New Bottom Plate_v4 (Autodesk Fusion 360 design; units mm, degrees)
Autodesk Fusion 360 part; units mm, degrees
note: some values were not read from the file. Set by a fixed rule: which sketch regions a step uses.
sketch "Reference" plane through (0, 0, 0) normal (0, 0, 1) x (1, 0, 0)
  line L0 (298.2751, -95.25) -> (298.2751, -113.3)
  line L1 (298.275, 1) -> (298.275, -57.15)
  line L2 (298.275, -57.15) -> (298.275, -57.15)
  line L3 (304.5217, -115.3) -> (303.775, 3)
  line L4 (179.47, 0) -> (290.235, 0)
  line L5 (290.2351, -112.3) -> (230.642, -112.3)
  line L6 (290.235, 1) -> (298.275, 1)
  line L7 (290.235, 0) -> (298.275, 0)
  line L8 (290.2351, -112.3) -> (298.2751, -112.3)
  arc A0 (302.0217, -117.8) -> (304.5217, -115.3) centre (302.0374, -115.3157) ccw
  line L9 (298.2751, -57.15) -> (298.2751, -74.2)
  line L10 (171.43, 0) -> (171.43, 1)
  line L11 (230.642, -112.3) -> (230.642, -113.3)
  line L12 (222.602, -113.3) -> (222.602, -112.3)
  arc A1 (303.775, 3) -> (301.275, 5.5) centre (301.275, 3) ccw
  line L13 (-28.337, -112.3) -> (-29.3375, -112.3)
  line L14 (-28.3375, 1.5) -> (-28.3375, 3)
  line L15 (-28.337, 1.5) -> (-6.3413, 1.5)
  line L16 (230.642, -112.3) -> (230.642, -113.3)
  line L17 (230.642, -113.3) -> (222.602, -113.3)
  line L18 (-36.12, -117.7958) -> (-31.338, -117.8)
  line L19 (222.602, -113.3) -> (222.602, -112.3)
  line L20 (-28.337, -113.3) -> (-28.337, -112.3)
  line L21 (-29.3375, -113.3) -> (-29.338, -113.3)
  arc A2 (-38.6178, -115.2937) -> (-36.12, -117.7958) centre (-36.1178, -115.2958) ccw
  line L22 (57.336, -112.3) -> (-20.297, -112.3)
  line L23 (8.02, 1) -> (8.02, 0)
  line L24 (-29.3375, -112.3) -> (-29.3375, -113.3)
  line L25 (-33.0995, -112.3) -> (-33.0995, 1.5)
  line L26 (-29.338, -112.3) -> (-33.0995, -112.3)
  line L27 (57.336, -113.3) -> (57.336, -112.3)
  line L28 (-20.297, -113.3) -> (-28.337, -113.3)
  line L29 (-29.338, -113.3) -> (-29.338, -112.3)
  line L30 (-20.297, -112.3) -> (-20.297, -113.3)
  line L31 (301.275, 5.5) -> (-36.0995, 5.5)
  line L32 (-38.5995, -94.25) -> (-38.6178, -115.2937)
  line L33 (298.2751, -76.2) -> (298.2751, -93.25)
  line L34 (298.275, -95.25) -> (298.275, -95.25)
  line L35 (298.275, -76.2) -> (298.275, -76.2)
  line L36 (-6.3413, 1.5) -> (-6.3413, 0)
  line L37 (-38.5995, 3) -> (-38.5995, -94.25)
  arc A3 (303.775, 3) -> (301.275, 5.5) centre (301.275, 3) ccw
  line L38 (298.2751, -74.2) -> (298.275, -74.2)
  line L39 (-28.337, 3) -> (-28.337, 1.5)
  line L40 (-33.0995, 1.5) -> (-28.3375, 1.5)
  line L41 (-0.02, 0) -> (-0.02, 1)
  arc A4 (-36.0995, 5.5) -> (-38.5995, 3) centre (-36.0995, 3) ccw
  line L42 (-31.338, -117.8) -> (302.0217, -117.8)
  line L43 (-6.3413, 0) -> (-0.02, 0)
  line L44 (298.275, -57.15) -> (298.275, -57.15)
  line L45 (-0.02, 1) -> (8.02, 1)
  line L46 (8.02, 0) -> (171.43, 0)
  line L47 (-28.3375, 3) -> (-28.337, 3)
  line L48 (290.235, 0) -> (290.235, 1)
  line L49 (290.235, 1) -> (298.275, 1)
  line L50 (298.2751, -57.15) -> (298.2751, -74.2)
  line L51 (298.275, 1) -> (298.275, -57.15)
  line L52 (222.602, -112.3) -> (65.376, -112.3)
  line L53 (-33.0995, -112.3) -> (-33.0995, 1.5)
  line L54 (301.275, 5.5) -> (-36.0995, 5.5)
  line L55 (-31.338, -117.8) -> (302.0217, -117.8)
  line L56 (57.336, -112.3) -> (-20.297, -112.3)
  line L57 (8.02, 0) -> (171.43, 0)
  line L58 (290.2351, -112.3) -> (230.642, -112.3)
  line L59 (298.2751, -95.25) -> (298.2751, -113.3)
  line L60 (298.275, -76.2) -> (298.275, -76.2)
  line L61 (298.275, -74.2) -> (298.275, -76.2)
  line L62 (298.2751, -76.2) -> (298.2751, -93.25)
  line L63 (298.2751, -93.25) -> (298.275, -93.25)
  line L64 (298.275, -93.25) -> (298.275, -95.25)
  line L65 (290.2351, -113.3) -> (290.2351, -112.3)
  arc A5 (302.0217, -117.8) -> (304.5217, -115.3) centre (302.0374, -115.3157) ccw
  line L66 (179.47, 0) -> (290.235, 0)
  line L67 (298.2751, -113.3) -> (290.2351, -113.3)
  line L68 (304.5217, -115.3) -> (303.775, 3)
  line L69 (298.275, -95.25) -> (298.275, -95.25)
  line L70 (57.336, -113.3) -> (57.336, -112.3)
  line L71 (65.376, -113.3) -> (57.336, -113.3)
  line L72 (-29.338, -113.3) -> (-29.338, -112.3)
  line L73 (-6.3413, 1.5) -> (-6.3413, 0)
  line L74 (-29.3375, -113.3) -> (-29.338, -113.3)
  line L75 (-29.3375, -112.3) -> (-29.3375, -113.3)
  line L76 (-28.3375, 1.5) -> (-28.3375, 3)
  line L77 (-28.337, 1.5) -> (-6.3413, 1.5)
  line L78 (-28.337, -112.3) -> (-29.3375, -112.3)
  line L79 (-28.337, -113.3) -> (-28.337, -112.3)
  line L80 (-28.3375, 3) -> (-28.337, 3)
  line L81 (-20.297, -113.3) -> (-28.337, -113.3)
  line L82 (65.376, -112.3) -> (65.376, -113.3)
  line L83 (-20.297, -112.3) -> (-20.297, -113.3)
  line L84 (-29.338, -112.3) -> (-33.0995, -112.3)
  line L85 (8.02, 1) -> (8.02, 0)
  line L86 (-28.337, 3) -> (-28.337, 1.5)
  arc A6 (-38.6178, -115.2937) -> (-36.12, -117.7958) centre (-36.1178, -115.2958) ccw
  line L87 (-38.5995, -94.25) -> (-38.6178, -115.2937)
  line L88 (-38.5995, 3) -> (-38.5995, -94.25)
  line L89 (-0.02, 0) -> (-0.02, 1)
  line L90 (-33.0995, 1.5) -> (-28.3375, 1.5)
  line L91 (-6.3413, 0) -> (-0.02, 0)
  arc A7 (-36.0995, 5.5) -> (-38.5995, 3) centre (-36.0995, 3) ccw
  line L92 (-0.02, 1) -> (8.02, 1)
  line L93 (-36.12, -117.7958) -> (-31.338, -117.8)
  line L94 (298.275, -93.25) -> (298.275, -95.25)
  line L95 (298.2751, -113.3) -> (290.2351, -113.3)
  line L96 (290.2351, -113.3) -> (290.2351, -112.3)
  line L97 (298.2751, -93.25) -> (298.275, -93.25)
  line L98 (298.275, -74.2) -> (298.275, -76.2)
  line L99 (298.2751, -74.2) -> (298.275, -74.2)
  line L100 (290.235, 0) -> (290.235, 1)
  line L101 (179.47, 1) -> (179.47, 0)
  line L102 (230.642, -113.3) -> (222.602, -113.3)
  line L103 (179.47, 1) -> (179.47, 0)
  line L104 (171.43, 1) -> (179.47, 1)
  line L105 (222.602, -112.3) -> (65.376, -112.3)
  line L106 (65.376, -112.3) -> (65.376, -113.3)
  line L107 (65.376, -113.3) -> (57.336, -113.3)
  line L108 (171.43, 0) -> (171.43, 1)
  line L109 (171.43, 1) -> (179.47, 1)
  dimension "d29" = 5.5
  dimension "d30" = 5.5
  dimension "d31" = 6.2339
  dimension "d32" = 5.5125
  dimension "d33" = 5.5
  dimension "d34" = 6.2276
  dimension "d35" = 5.5188
  constraint coincident L5.start L8.start
  constraint perpendicular L0 L8
  constraint coincident L8.end L59
  constraint coincident L4.end L7.start
  constraint perpendicular L7 L48
  constraint coincident L7.end L51
  measures "d29" distance of L42 L58
  measures "d30" distance of L4 L31
  measures "d31" distance of L0.end L3
  measures "d32" distance of L1.start L3
  measures "d33" distance of L25 L37
  measures "d34" distance of L8.end L3
  measures "d35" distance of L7.end L68
sketch "FlatPlateSketch" plane through (0, 0, 0) normal (0, 0, 1) x (1, 0, 0)
  line L0 (298.2751, -95.25) -> (298.2751, -113.3)
  line L1 (298.275, 1) -> (298.275, -57.15)
  line L2 (298.275, -57.15) -> (298.275, -57.15)
  line L3 (304.5217, -115.3) -> (303.775, 3)
  line L4 (179.47, 0) -> (290.235, 0)
  line L5 (290.2351, -112.3) -> (230.642, -112.3)
  line L6 (290.235, 1) -> (298.275, 1)
  line L7 (290.235, 0) -> (298.275, 0)
  line L8 (290.2351, -112.3) -> (298.2751, -112.3)
  arc A0 (302.0217, -117.8) -> (304.5217, -115.3) centre (302.0374, -115.3157) ccw
  line L9 (298.2751, -57.15) -> (298.2751, -74.2)
  line L10 (171.43, 0) -> (171.43, 1)
  line L11 (230.642, -112.3) -> (230.642, -113.3)
  line L12 (222.602, -113.3) -> (222.602, -112.3)
  arc A1 (303.775, 3) -> (301.275, 5.5) centre (301.275, 3) ccw
  line L13 (-28.337, -112.3) -> (-29.3375, -112.3)
  line L14 (-28.3375, 1.5) -> (-28.3375, 3)
  line L15 (-28.337, 1.5) -> (-6.3413, 1.5)
  line L16 (230.642, -112.3) -> (230.642, -113.3)
  line L17 (230.642, -113.3) -> (222.602, -113.3)
  line L18 (-36.12, -117.7958) -> (-31.338, -117.8)
  line L19 (222.602, -113.3) -> (222.602, -112.3)
  line L20 (-28.337, -113.3) -> (-28.337, -112.3)
  line L21 (-29.3375, -113.3) -> (-29.338, -113.3)
  arc A2 (-38.6178, -115.2937) -> (-36.12, -117.7958) centre (-36.1178, -115.2958) ccw
  line L22 (57.336, -112.3) -> (-20.297, -112.3)
  line L23 (8.02, 1) -> (8.02, 0)
  line L24 (-29.3375, -112.3) -> (-29.3375, -113.3)
  line L25 (-33.0995, -112.3) -> (-33.0995, 1.5)
  line L26 (-29.338, -112.3) -> (-33.0995, -112.3)
  line L27 (57.336, -113.3) -> (57.336, -112.3)
  line L28 (-20.297, -113.3) -> (-28.337, -113.3)
  line L29 (-29.338, -113.3) -> (-29.338, -112.3)
  line L30 (-20.297, -112.3) -> (-20.297, -113.3)
  line L31 (301.275, 5.5) -> (-36.0995, 5.5)
  line L32 (-38.5995, -94.25) -> (-38.6178, -115.2937)
  line L33 (298.2751, -76.2) -> (298.2751, -93.25)
  line L34 (298.275, -95.25) -> (298.275, -95.25)
  line L35 (298.275, -76.2) -> (298.275, -76.2)
  line L36 (-6.3413, 1.5) -> (-6.3413, 0)
  line L37 (-38.5995, 3) -> (-38.5995, -94.25)
  arc A3 (303.775, 3) -> (301.275, 5.5) centre (301.275, 3) ccw
  line L38 (298.2751, -74.2) -> (298.275, -74.2)
  line L39 (-28.337, 3) -> (-28.337, 1.5)
  line L40 (-33.0995, 1.5) -> (-28.3375, 1.5)
  line L41 (-0.02, 0) -> (-0.02, 1)
  arc A4 (-36.0995, 5.5) -> (-38.5995, 3) centre (-36.0995, 3) ccw
  line L42 (-31.338, -117.8) -> (302.0217, -117.8)
  line L43 (-6.3413, 0) -> (-0.02, 0)
  line L44 (298.275, -57.15) -> (298.275, -57.15)
  line L45 (-0.02, 1) -> (8.02, 1)
  line L46 (8.02, 0) -> (171.43, 0)
  line L47 (-28.3375, 3) -> (-28.337, 3)
  line L48 (290.235, 0) -> (290.235, 1)
  line L49 (290.235, 1) -> (298.275, 1)
  line L50 (298.2751, -57.15) -> (298.2751, -74.2)
  line L51 (298.275, 1) -> (298.275, -57.15)
  line L52 (222.602, -112.3) -> (65.376, -112.3)
  line L53 (-33.0995, -112.3) -> (-33.0995, 1.5)
  line L54 (301.275, 5.5) -> (-36.0995, 5.5)
  line L55 (-31.338, -117.8) -> (302.0217, -117.8)
  line L56 (57.336, -112.3) -> (-20.297, -112.3)
  line L57 (8.02, 0) -> (171.43, 0)
  line L58 (290.2351, -112.3) -> (230.642, -112.3)
  line L59 (298.2751, -95.25) -> (298.2751, -113.3)
  line L60 (298.275, -76.2) -> (298.275, -76.2)
  line L61 (298.275, -74.2) -> (298.275, -76.2)
  line L62 (298.2751, -76.2) -> (298.2751, -93.25)
  line L63 (298.2751, -93.25) -> (298.275, -93.25)
  line L64 (298.275, -93.25) -> (298.275, -95.25)
  line L65 (290.2351, -113.3) -> (290.2351, -112.3)
  arc A5 (302.0217, -117.8) -> (304.5217, -115.3) centre (302.0374, -115.3157) ccw
  line L66 (179.47, 0) -> (290.235, 0)
  line L67 (298.2751, -113.3) -> (290.2351, -113.3)
  line L68 (304.5217, -115.3) -> (303.775, 3)
  line L69 (298.275, -95.25) -> (298.275, -95.25)
  line L70 (57.336, -113.3) -> (57.336, -112.3)
  line L71 (65.376, -113.3) -> (57.336, -113.3)
  line L72 (-29.338, -113.3) -> (-29.338, -112.3)
  line L73 (-6.3413, 1.5) -> (-6.3413, 0)
  line L74 (-29.3375, -113.3) -> (-29.338, -113.3)
  line L75 (-29.3375, -112.3) -> (-29.3375, -113.3)
  line L76 (-28.3375, 1.5) -> (-28.3375, 3)
  line L77 (-28.337, 1.5) -> (-6.3413, 1.5)
  line L78 (-28.337, -112.3) -> (-29.3375, -112.3)
  line L79 (-28.337, -113.3) -> (-28.337, -112.3)
  line L80 (-28.3375, 3) -> (-28.337, 3)
  line L81 (-20.297, -113.3) -> (-28.337, -113.3)
  line L82 (65.376, -112.3) -> (65.376, -113.3)
  line L83 (-20.297, -112.3) -> (-20.297, -113.3)
  line L84 (-29.338, -112.3) -> (-33.0995, -112.3)
  line L85 (8.02, 1) -> (8.02, 0)
  line L86 (-28.337, 3) -> (-28.337, 1.5)
  arc A6 (-38.6178, -115.2937) -> (-36.12, -117.7958) centre (-36.1178, -115.2958) ccw
  line L87 (-38.5995, -94.25) -> (-38.6178, -115.2937)
  line L88 (-38.5995, 3) -> (-38.5995, -94.25)
  line L89 (-0.02, 0) -> (-0.02, 1)
  line L90 (-33.0995, 1.5) -> (-28.3375, 1.5)
  line L91 (-6.3413, 0) -> (-0.02, 0)
  arc A7 (-36.0995, 5.5) -> (-38.5995, 3) centre (-36.0995, 3) ccw
  line L92 (-0.02, 1) -> (8.02, 1)
  line L93 (-36.12, -117.7958) -> (-31.338, -117.8)
  line L94 (298.275, -93.25) -> (298.275, -95.25)
  line L95 (298.2751, -113.3) -> (290.2351, -113.3)
  line L96 (290.2351, -113.3) -> (290.2351, -112.3)
  line L97 (298.2751, -93.25) -> (298.275, -93.25)
  line L98 (298.275, -74.2) -> (298.275, -76.2)
  line L99 (298.2751, -74.2) -> (298.275, -74.2)
  line L100 (290.235, 0) -> (290.235, 1)
  line L101 (179.47, 1) -> (179.47, 0)
  line L102 (230.642, -113.3) -> (222.602, -113.3)
  line L103 (179.47, 1) -> (179.47, 0)
  line L104 (171.43, 1) -> (179.47, 1)
  line L105 (222.602, -112.3) -> (65.376, -112.3)
  line L106 (65.376, -112.3) -> (65.376, -113.3)
  line L107 (65.376, -113.3) -> (57.336, -113.3)
  line L108 (171.43, 0) -> (171.43, 1)
  line L109 (171.43, 1) -> (179.47, 1)
  dimension "d36" = 5.5
  dimension "d37" = 5.5
  dimension "d38" = 6.2339
  dimension "d39" = 5.5125
  dimension "d40" = 5.5
  dimension "d41" = 6.2276
  dimension "d42" = 5.5188
  constraint coincident L5.start L8.start
  constraint perpendicular L0 L8
  constraint coincident L8.end L59
  constraint coincident L4.end L7.start
  constraint perpendicular L7 L48
  constraint coincident L7.end L51
  measures "d36" distance of L42 L58
  measures "d37" distance of L4 L31
  measures "d38" distance of L0.end L3
  measures "d39" distance of L1.start L3
  measures "d40" distance of L25 L37
  measures "d41" distance of L8.end L3
  measures "d42" distance of L7.end L68
sketch "LipSketch" plane through (0, 0, 0) normal (0, 0, 1) x (1, 0, 0)
  line L0 (298.2751, -95.25) -> (298.2751, -113.3)
  line L1 (298.275, 1) -> (298.275, -57.15)
  line L2 (298.275, -57.15) -> (298.275, -57.15)
  line L3 (304.5217, -115.3) -> (303.775, 3)
  line L4 (179.47, 0) -> (290.235, 0)
  line L5 (290.2351, -112.3) -> (230.642, -112.3)
  line L6 (290.235, 1) -> (298.275, 1)
  line L7 (290.235, 0) -> (298.275, 0)
  line L8 (290.2351, -112.3) -> (298.2751, -112.3)
  arc A0 (302.0217, -117.8) -> (304.5217, -115.3) centre (302.0374, -115.3157) ccw
  line L9 (298.2751, -57.15) -> (298.2751, -74.2)
  line L10 (171.43, 0) -> (171.43, 1)
  line L11 (230.642, -112.3) -> (230.642, -113.3)
  line L12 (222.602, -113.3) -> (222.602, -112.3)
  arc A1 (303.775, 3) -> (301.275, 5.5) centre (301.275, 3) ccw
  line L13 (-28.337, -112.3) -> (-29.3375, -112.3)
  line L14 (-28.3375, 1.5) -> (-28.3375, 3)
  line L15 (-28.337, 1.5) -> (-6.3413, 1.5)
  line L16 (230.642, -112.3) -> (230.642, -113.3)
  line L17 (230.642, -113.3) -> (222.602, -113.3)
  line L18 (-36.12, -117.7958) -> (-31.338, -117.8)
  line L19 (222.602, -113.3) -> (222.602, -112.3)
  line L20 (-28.337, -113.3) -> (-28.337, -112.3)
  line L21 (-29.3375, -113.3) -> (-29.338, -113.3)
  arc A2 (-38.6178, -115.2937) -> (-36.12, -117.7958) centre (-36.1178, -115.2958) ccw
  line L22 (57.336, -112.3) -> (-20.297, -112.3)
  line L23 (8.02, 1) -> (8.02, 0)
  line L24 (-29.3375, -112.3) -> (-29.3375, -113.3)
  line L25 (-33.0995, -112.3) -> (-33.0995, 1.5)
  line L26 (-29.338, -112.3) -> (-33.0995, -112.3)
  line L27 (57.336, -113.3) -> (57.336, -112.3)
  line L28 (-20.297, -113.3) -> (-28.337, -113.3)
  line L29 (-29.338, -113.3) -> (-29.338, -112.3)
  line L30 (-20.297, -112.3) -> (-20.297, -113.3)
  line L31 (301.275, 5.5) -> (-36.0995, 5.5)
  line L32 (-38.5995, -94.25) -> (-38.6178, -115.2937)
  line L33 (298.2751, -76.2) -> (298.2751, -93.25)
  line L34 (298.275, -95.25) -> (298.275, -95.25)
  line L35 (298.275, -76.2) -> (298.275, -76.2)
  line L36 (-6.3413, 1.5) -> (-6.3413, 0)
  line L37 (-38.5995, 3) -> (-38.5995, -94.25)
  arc A3 (303.775, 3) -> (301.275, 5.5) centre (301.275, 3) ccw
  line L38 (298.2751, -74.2) -> (298.275, -74.2)
  line L39 (-28.337, 3) -> (-28.337, 1.5)
  line L40 (-33.0995, 1.5) -> (-28.3375, 1.5)
  line L41 (-0.02, 0) -> (-0.02, 1)
  arc A4 (-36.0995, 5.5) -> (-38.5995, 3) centre (-36.0995, 3) ccw
  line L42 (-31.338, -117.8) -> (302.0217, -117.8)
  line L43 (-6.3413, 0) -> (-0.02, 0)
  line L44 (298.275, -57.15) -> (298.275, -57.15)
  line L45 (-0.02, 1) -> (8.02, 1)
  line L46 (8.02, 0) -> (171.43, 0)
  line L47 (-28.3375, 3) -> (-28.337, 3)
  line L48 (290.235, 0) -> (290.235, 1)
  line L49 (290.235, 1) -> (298.275, 1)
  line L50 (298.2751, -57.15) -> (298.2751, -74.2)
  line L51 (298.275, 1) -> (298.275, -57.15)
  line L52 (222.602, -112.3) -> (65.376, -112.3)
  line L53 (-33.0995, -112.3) -> (-33.0995, 1.5)
  line L54 (301.275, 5.5) -> (-36.0995, 5.5)
  line L55 (-31.338, -117.8) -> (302.0217, -117.8)
  line L56 (57.336, -112.3) -> (-20.297, -112.3)
  line L57 (8.02, 0) -> (171.43, 0)
  line L58 (290.2351, -112.3) -> (230.642, -112.3)
  line L59 (298.2751, -95.25) -> (298.2751, -113.3)
  line L60 (298.275, -76.2) -> (298.275, -76.2)
  line L61 (298.275, -74.2) -> (298.275, -76.2)
  line L62 (298.2751, -76.2) -> (298.2751, -93.25)
  line L63 (298.2751, -93.25) -> (298.275, -93.25)
  line L64 (298.275, -93.25) -> (298.275, -95.25)
  line L65 (290.2351, -113.3) -> (290.2351, -112.3)
  arc A5 (302.0217, -117.8) -> (304.5217, -115.3) centre (302.0374, -115.3157) ccw
  line L66 (179.47, 0) -> (290.235, 0)
  line L67 (298.2751, -113.3) -> (290.2351, -113.3)
  line L68 (304.5217, -115.3) -> (303.775, 3)
  line L69 (298.275, -95.25) -> (298.275, -95.25)
  line L70 (57.336, -113.3) -> (57.336, -112.3)
  line L71 (65.376, -113.3) -> (57.336, -113.3)
  line L72 (-29.338, -113.3) -> (-29.338, -112.3)
  line L73 (-6.3413, 1.5) -> (-6.3413, 0)
  line L74 (-29.3375, -113.3) -> (-29.338, -113.3)
  line L75 (-29.3375, -112.3) -> (-29.3375, -113.3)
  line L76 (-28.3375, 1.5) -> (-28.3375, 3)
  line L77 (-28.337, 1.5) -> (-6.3413, 1.5)
  line L78 (-28.337, -112.3) -> (-29.3375, -112.3)
  line L79 (-28.337, -113.3) -> (-28.337, -112.3)
  line L80 (-28.3375, 3) -> (-28.337, 3)
  line L81 (-20.297, -113.3) -> (-28.337, -113.3)
  line L82 (65.376, -112.3) -> (65.376, -113.3)
  line L83 (-20.297, -112.3) -> (-20.297, -113.3)
  line L84 (-29.338, -112.3) -> (-33.0995, -112.3)
  line L85 (8.02, 1) -> (8.02, 0)
  line L86 (-28.337, 3) -> (-28.337, 1.5)
  arc A6 (-38.6178, -115.2937) -> (-36.12, -117.7958) centre (-36.1178, -115.2958) ccw
  line L87 (-38.5995, -94.25) -> (-38.6178, -115.2937)
  line L88 (-38.5995, 3) -> (-38.5995, -94.25)
  line L89 (-0.02, 0) -> (-0.02, 1)
  line L90 (-33.0995, 1.5) -> (-28.3375, 1.5)
  line L91 (-6.3413, 0) -> (-0.02, 0)
  arc A7 (-36.0995, 5.5) -> (-38.5995, 3) centre (-36.0995, 3) ccw
  line L92 (-0.02, 1) -> (8.02, 1)
  line L93 (-36.12, -117.7958) -> (-31.338, -117.8)
  line L94 (298.275, -93.25) -> (298.275, -95.25)
  line L95 (298.2751, -113.3) -> (290.2351, -113.3)
  line L96 (290.2351, -113.3) -> (290.2351, -112.3)
  line L97 (298.2751, -93.25) -> (298.275, -93.25)
  line L98 (298.275, -74.2) -> (298.275, -76.2)
  line L99 (298.2751, -74.2) -> (298.275, -74.2)
  line L100 (290.235, 0) -> (290.235, 1)
  line L101 (179.47, 1) -> (179.47, 0)
  line L102 (230.642, -113.3) -> (222.602, -113.3)
  line L103 (179.47, 1) -> (179.47, 0)
  line L104 (171.43, 1) -> (179.47, 1)
  line L105 (222.602, -112.3) -> (65.376, -112.3)
  line L106 (65.376, -112.3) -> (65.376, -113.3)
  line L107 (65.376, -113.3) -> (57.336, -113.3)
  line L108 (171.43, 0) -> (171.43, 1)
  line L109 (171.43, 1) -> (179.47, 1)
  line L110 (290.235, 0) -> (290.235, -0.5) construction
  line L111 (298.275, -3.3243) -> (297.775, -3.3243) construction
  line L112 (286.7003, -112.3) -> (286.7003, -111.8) construction
  line L113 (298.2751, -110.893) -> (297.7751, -110.893) construction
  line L114 (286.7003, -111.8) -> (297.7751, -111.8)
  line L115 (297.7751, -110.893) -> (297.7751, -111.8)
  line L116 (297.7751, -110.893) -> (297.7751, -0.5)
  line L117 (290.235, -0.5) -> (297.7751, -0.5)
  line L118 (290.235, -0.5) -> (-27.25, -0.5)
  line L119 (-33.0995, -0.5) -> (-32.5995, -0.5) construction
  line L120 (-32.5995, -0.5) -> (-27.25, -0.5)
  line L121 (-33.0995, -111.8) -> (-32.5995, -111.8) construction
  line L122 (-32.5995, -111.8) -> (-32.5995, -0.5)
  line L123 (286.7003, -111.8) -> (-31.0685, -111.8)
  line L124 (-31.0685, -111.8) -> (-32.5995, -111.8)
  line L125 (-32.5995, -0.5) -> (-30.5995, -0.5)
  line L126 (-30.5995, -0.5) -> (-30.5995, -2.5) construction
  line L127 (-32.5995, -2.5) -> (-32.5995, -0.5)
  line L128 (-32.5995, -111.8) -> (-30.5995, -111.8)
  line L129 (-30.5995, -111.8) -> (-30.5995, -109.8) construction
  line L130 (-30.5995, -109.8) -> (-32.5995, -109.8) construction
  line L131 (-32.5995, -109.8) -> (-32.5995, -111.8)
  line L132 (297.7751, -111.8) -> (295.7751, -111.8)
  line L133 (295.7751, -111.8) -> (295.7751, -109.8) construction
  line L134 (295.7751, -109.8) -> (297.7751, -109.8) construction
  line L135 (297.7751, -109.8) -> (297.7751, -111.8)
  line L136 (297.7751, -0.5) -> (295.7751, -0.5)
  line L137 (295.7751, -0.5) -> (295.7751, -2.5) construction
  line L138 (295.7751, -2.5) -> (297.7751, -2.5) construction
  line L139 (297.7751, -2.5) -> (297.7751, -0.5)
  line L140 (295.7751, -2.5) -> (-30.5995, -2.5)
  line L141 (-30.5995, -2.5) -> (-30.5995, -109.8)
  line L142 (-30.5995, -109.8) -> (295.7751, -109.8)
  line L143 (295.7751, -109.8) -> (295.7751, -2.5)
  dimension "d45" = 5.5
  dimension "d46" = 5.5
  dimension "d47" = 6.2339
  dimension "d48" = 5.5125
  dimension "d49" = 5.5
  dimension "d50" = 6.2276
  dimension "d51" = 5.5188
  dimension "d68" = 0.5
  dimension "d69" = 0.5
  dimension "d70" = 0.5
  dimension "d71" = 0.5
  dimension "d72" = 0.5
  dimension "d73" = 0.5
  dimension "d74" = 2
  dimension "d75" = 2
  dimension "d76" = 2
  dimension "d77" = 2
  dimension "d78" = 2
  dimension "d79" = 2
  dimension "d80" = 2
  dimension "d81" = 2
  constraint coincident L5.start L8.start
  constraint perpendicular L0 L8
  constraint coincident L8.end L59
  constraint coincident L4.end L7.start
  constraint perpendicular L7 L48
  constraint coincident L7.end L51
  constraint perpendicular L7 L110
  constraint coincident L1 L111.start
  constraint perpendicular L1 L111
  constraint coincident L58 L112.start
  constraint perpendicular L58 L112
  constraint coincident L59 L113.start
  constraint perpendicular L59 L113
  constraint perpendicular L0 L114
  constraint perpendicular L113 L115
  constraint perpendicular L6 L116
  constraint perpendicular L110 L117
  constraint perpendicular L25 L118
  constraint coincident L25 L119.start
  constraint perpendicular L25 L119
  constraint parallel L119 L120
  constraint perpendicular L25 L123
  constraint coincident L25 L121.start
  constraint perpendicular L53 L121
  constraint horizontal L125
  constraint vertical L126
  constraint vertical L127
  constraint horizontal L128
  constraint vertical L129
  constraint horizontal L130
  constraint vertical L131
  constraint horizontal L132
  constraint vertical L133
  constraint horizontal L134
  constraint vertical L135
  constraint horizontal L136
  constraint vertical L137
  constraint horizontal L138
  constraint vertical L139
  constraint perpendicular L126 L140
  constraint perpendicular L130 L141
  constraint perpendicular L133 L142
  constraint perpendicular L138 L143
  measures "d45" distance of L42 L58
  measures "d46" distance of L4 L31
  measures "d47" distance of L0.end L3
  measures "d48" distance of L1.start L3
  measures "d49" distance of L25 L37
  measures "d50" distance of L8.end L3
  measures "d51" distance of L7.end L68
  measures "d68" distance of L4.end L110.end
  measures "d69" distance of L111.start L111.end
  measures "d70" distance of L112.start L112.end
  measures "d71" distance of L113.start L113.end
  measures "d72" distance of L119.start L119.end
  measures "d73" distance of L121.start L121.end
  measures "d74" distance of L119.end L125.end
  measures "d75" distance of L119.end L127.start
  measures "d76" distance of L121.end L128.end
  measures "d77" distance of L121.end L130.end
  measures "d78" distance of L114.end L132.end
  measures "d79" distance of L114.end L134.end
  measures "d80" distance of L116.end L136.end
  measures "d81" distance of L116.end L138.end
extrude "Extrude4" add sketch "FlatPlateSketch" against normal blind 1 contours L0 L1 L4 L5 L7 L8 L9 L10 L11 L12 L13 L15 L16 L17 L19 L20 L22 L23 L25 L26 L27 L28 L30 L33 L36 L40 L41 L43 L45 L46 L50 L51 L52 L53 L56 L57 L58 L59 L61 L62 L64 L66 L70 L71 L73 L77 L78 L79 L81 L82 L83 L84 L85 L89 L90 L91 L92 L94 L98 L101 L102 L103 L104 L105 L106 L107 L108 L109 | L0 L8 L59 L65 L67 L95 L96 | L1 L6 L7 L48 L49 L51 L100 | L3 A0 A1 L18 A2 L31 L32 L37 A3 A4 L42 L54 L55 A5 L68 A6 L87 L88 A7 L93
sketch "Sketch8" plane through (0, 0, 0) normal (0, 0, 1) x (1, 0, 0)
  line L0 (298.2751, -95.25) -> (298.2751, -113.3)
  line L1 (298.275, 1) -> (298.275, -57.15)
  line L2 (298.275, -57.15) -> (298.275, -57.15)
  line L3 (304.5217, -115.3) -> (303.775, 3)
  line L4 (179.47, 0) -> (290.235, 0)
  line L5 (290.2351, -112.3) -> (230.642, -112.3)
  line L6 (290.235, 1) -> (298.275, 1)
  line L7 (290.235, 0) -> (298.275, 0)
  line L8 (290.2351, -112.3) -> (298.2751, -112.3)
  arc A0 (302.0217, -117.8) -> (304.5217, -115.3) centre (302.0374, -115.3157) ccw
  line L9 (298.2751, -57.15) -> (298.2751, -74.2)
  line L10 (171.43, 0) -> (171.43, 1)
  line L11 (230.642, -112.3) -> (230.642, -113.3)
  line L12 (222.602, -113.3) -> (222.602, -112.3)
  arc A1 (303.775, 3) -> (301.275, 5.5) centre (301.275, 3) ccw
  line L13 (-28.337, -112.3) -> (-29.3375, -112.3)
  line L14 (-28.3375, 1.5) -> (-28.3375, 3)
  line L15 (-28.337, 1.5) -> (-6.3413, 1.5)
  line L16 (230.642, -112.3) -> (230.642, -113.3)
  line L17 (230.642, -113.3) -> (222.602, -113.3)
  line L18 (-36.12, -117.7958) -> (-31.338, -117.8)
  line L19 (222.602, -113.3) -> (222.602, -112.3)
  line L20 (-28.337, -113.3) -> (-28.337, -112.3)
  line L21 (-29.3375, -113.3) -> (-29.338, -113.3)
  arc A2 (-38.6178, -115.2937) -> (-36.12, -117.7958) centre (-36.1178, -115.2958) ccw
  line L22 (57.336, -112.3) -> (-20.297, -112.3)
  line L23 (8.02, 1) -> (8.02, 0)
  line L24 (-29.3375, -112.3) -> (-29.3375, -113.3)
  line L25 (-33.0995, -112.3) -> (-33.0995, 1.5)
  line L26 (-29.338, -112.3) -> (-33.0995, -112.3)
  line L27 (57.336, -113.3) -> (57.336, -112.3)
  line L28 (-20.297, -113.3) -> (-28.337, -113.3)
  line L29 (-29.338, -113.3) -> (-29.338, -112.3)
  line L30 (-20.297, -112.3) -> (-20.297, -113.3)
  line L31 (301.275, 5.5) -> (-36.0995, 5.5)
  line L32 (-38.5995, -94.25) -> (-38.6178, -115.2937)
  line L33 (298.2751, -76.2) -> (298.2751, -93.25)
  line L34 (298.275, -95.25) -> (298.275, -95.25)
  line L35 (298.275, -76.2) -> (298.275, -76.2)
  line L36 (-6.3413, 1.5) -> (-6.3413, 0)
  line L37 (-38.5995, 3) -> (-38.5995, -94.25)
  arc A3 (303.775, 3) -> (301.275, 5.5) centre (301.275, 3) ccw
  line L38 (298.2751, -74.2) -> (298.275, -74.2)
  line L39 (-28.337, 3) -> (-28.337, 1.5)
  line L40 (-33.0995, 1.5) -> (-28.3375, 1.5)
  line L41 (-0.02, 0) -> (-0.02, 1)
  arc A4 (-36.0995, 5.5) -> (-38.5995, 3) centre (-36.0995, 3) ccw
  line L42 (-31.338, -117.8) -> (302.0217, -117.8)
  line L43 (-6.3413, 0) -> (-0.02, 0)
  line L44 (298.275, -57.15) -> (298.275, -57.15)
  line L45 (-0.02, 1) -> (8.02, 1)
  line L46 (8.02, 0) -> (171.43, 0)
  line L47 (-28.3375, 3) -> (-28.337, 3)
  line L48 (290.235, 0) -> (290.235, 1)
  line L49 (290.235, 1) -> (298.275, 1)
  line L50 (298.2751, -57.15) -> (298.2751, -74.2)
  line L51 (298.275, 1) -> (298.275, -57.15)
  line L52 (222.602, -112.3) -> (65.376, -112.3)
  line L53 (-33.0995, -112.3) -> (-33.0995, 1.5)
  line L54 (301.275, 5.5) -> (-36.0995, 5.5)
  line L55 (-31.338, -117.8) -> (302.0217, -117.8)
  line L56 (57.336, -112.3) -> (-20.297, -112.3)
  line L57 (8.02, 0) -> (171.43, 0)
  line L58 (290.2351, -112.3) -> (230.642, -112.3)
  line L59 (298.2751, -95.25) -> (298.2751, -113.3)
  line L60 (298.275, -76.2) -> (298.275, -76.2)
  line L61 (298.275, -74.2) -> (298.275, -76.2)
  line L62 (298.2751, -76.2) -> (298.2751, -93.25)
  line L63 (298.2751, -93.25) -> (298.275, -93.25)
  line L64 (298.275, -93.25) -> (298.275, -95.25)
  line L65 (290.2351, -113.3) -> (290.2351, -112.3)
  arc A5 (302.0217, -117.8) -> (304.5217, -115.3) centre (302.0374, -115.3157) ccw
  line L66 (179.47, 0) -> (290.235, 0)
  line L67 (298.2751, -113.3) -> (290.2351, -113.3)
  line L68 (304.5217, -115.3) -> (303.775, 3)
  line L69 (298.275, -95.25) -> (298.275, -95.25)
  line L70 (57.336, -113.3) -> (57.336, -112.3)
  line L71 (65.376, -113.3) -> (57.336, -113.3)
  line L72 (-29.338, -113.3) -> (-29.338, -112.3)
  line L73 (-6.3413, 1.5) -> (-6.3413, 0)
  line L74 (-29.3375, -113.3) -> (-29.338, -113.3)
  line L75 (-29.3375, -112.3) -> (-29.3375, -113.3)
  line L76 (-28.3375, 1.5) -> (-28.3375, 3)
  line L77 (-28.337, 1.5) -> (-6.3413, 1.5)
  line L78 (-28.337, -112.3) -> (-29.3375, -112.3)
  line L79 (-28.337, -113.3) -> (-28.337, -112.3)
  line L80 (-28.3375, 3) -> (-28.337, 3)
  line L81 (-20.297, -113.3) -> (-28.337, -113.3)
  line L82 (65.376, -112.3) -> (65.376, -113.3)
  line L83 (-20.297, -112.3) -> (-20.297, -113.3)
  line L84 (-29.338, -112.3) -> (-33.0995, -112.3)
  line L85 (8.02, 1) -> (8.02, 0)
  line L86 (-28.337, 3) -> (-28.337, 1.5)
  arc A6 (-38.6178, -115.2937) -> (-36.12, -117.7958) centre (-36.1178, -115.2958) ccw
  line L87 (-38.5995, -94.25) -> (-38.6178, -115.2937)
  line L88 (-38.5995, 3) -> (-38.5995, -94.25)
  line L89 (-0.02, 0) -> (-0.02, 1)
  line L90 (-33.0995, 1.5) -> (-28.3375, 1.5)
  line L91 (-6.3413, 0) -> (-0.02, 0)
  arc A7 (-36.0995, 5.5) -> (-38.5995, 3) centre (-36.0995, 3) ccw
  line L92 (-0.02, 1) -> (8.02, 1)
  line L93 (-36.12, -117.7958) -> (-31.338, -117.8)
  line L94 (298.275, -93.25) -> (298.275, -95.25)
  line L95 (298.2751, -113.3) -> (290.2351, -113.3)
  line L96 (290.2351, -113.3) -> (290.2351, -112.3)
  line L97 (298.2751, -93.25) -> (298.275, -93.25)
  line L98 (298.275, -74.2) -> (298.275, -76.2)
  line L99 (298.2751, -74.2) -> (298.275, -74.2)
  line L100 (290.235, 0) -> (290.235, 1)
  line L101 (179.47, 1) -> (179.47, 0)
  line L102 (230.642, -113.3) -> (222.602, -113.3)
  line L103 (179.47, 1) -> (179.47, 0)
  line L104 (171.43, 1) -> (179.47, 1)
  line L105 (222.602, -112.3) -> (65.376, -112.3)
  line L106 (65.376, -112.3) -> (65.376, -113.3)
  line L107 (65.376, -113.3) -> (57.336, -113.3)
  line L108 (171.43, 0) -> (171.43, 1)
  line L109 (171.43, 1) -> (179.47, 1)
  dimension "d54" = 5.5
  dimension "d55" = 5.5
  dimension "d56" = 6.2339
  dimension "d57" = 5.5125
  dimension "d58" = 5.5
  dimension "d59" = 6.2276
  dimension "d60" = 5.5188
  constraint coincident L5.start L8.start
  constraint perpendicular L0 L8
  constraint coincident L8.end L59
  constraint coincident L4.end L7.start
  constraint perpendicular L7 L48
  constraint coincident L7.end L51
  measures "d54" distance of L42 L58
  measures "d55" distance of L4 L31
  measures "d56" distance of L0.end L3
  measures "d57" distance of L1.start L3
  measures "d58" distance of L25 L37
  measures "d59" distance of L8.end L3
  measures "d60" distance of L7.end L68
extrude "LipExtrude" add sketch "LipSketch" along normal blind 2 contours L114 L115 L116 L117 L118 L120 L122 L123 L124 L125 L127 L128 L131 L132 L135 L136 L139
sketch "USBHoleSketch" plane through (0, 0, 2) normal (0, 0, 1) x (-1, 0, 0)
  line L0 (-295.7751, 2.5) -> (-295.7751, 109.8)
  line L1 (-295.7751, 109.8) -> (30.5995, 109.8)
  line L2 (30.5995, 109.8) -> (30.5995, 2.5)
  line L3 (30.5995, 2.5) -> (-295.7751, 2.5)
  line L4 (-297.7751, 111.8) -> (-297.7751, 0.5)
  line L5 (-297.7751, 0.5) -> (32.5995, 0.5)
  line L6 (32.5995, 0.5) -> (32.5995, 111.8)
  line L7 (32.5995, 111.8) -> (-297.7751, 111.8)
  line L8 (32.5995, 0.5) -> (-132.588, 0.5) construction
  line L9 (-132.588, 0.5) -> (-139.338, 0.5)
  line L10 (-139.338, 0.5) -> (-139.338, 2.5)
  line L11 (-139.338, 2.5) -> (-125.838, 2.5)
  line L12 (-125.838, 2.5) -> (-125.838, 0.5)
  line L13 (-125.838, 0.5) -> (-132.588, 0.5)
  dimension "d84" = 165.1875
  dimension "d85" = 6.75
  dimension "d86" = 13.5
  constraint coincident L5.end L6.start
  constraint perpendicular L4 L8
  constraint parallel L5 L9
  constraint coincident L3 L10.end
  constraint perpendicular L3 L10
  constraint perpendicular L10 L11
  constraint perpendicular L5 L12
  constraint coincident L5 L12.end
  measures "d84" distance of L5.end L8.end
  measures "d85" distance of L8.end L9.end
  measures "d86" distance of L10.end L11.end
extrude "Extrude6" cut sketch "USBHoleSketch" against normal blind 2 contours L3 L5 L9 L10 L11 L12 L13
sketch "Sketch9" plane through (0, 0, 0) normal (0, 0, 1) x (1, 0, 0)
  line L0 (298.2751, -95.25) -> (298.2751, -113.3)
  line L1 (298.275, 1) -> (298.275, -57.15)
  line L2 (298.275, -57.15) -> (298.275, -57.15)
  line L3 (304.5217, -115.3) -> (303.775, 3)
  line L4 (179.47, 0) -> (290.235, 0)
  line L5 (290.2351, -112.3) -> (230.642, -112.3)
  line L6 (290.235, 1) -> (298.275, 1)
  line L7 (290.235, 0) -> (298.275, 0)
  line L8 (290.2351, -112.3) -> (298.2751, -112.3)
  arc A0 (302.0217, -117.8) -> (304.5217, -115.3) centre (302.0374, -115.3157) ccw
  line L9 (298.2751, -57.15) -> (298.2751, -74.2)
  line L10 (171.43, 0) -> (171.43, 1)
  line L11 (230.642, -112.3) -> (230.642, -113.3)
  line L12 (222.602, -113.3) -> (222.602, -112.3)
  arc A1 (303.775, 3) -> (301.275, 5.5) centre (301.275, 3) ccw
  line L13 (-28.337, -112.3) -> (-29.3375, -112.3)
  line L14 (-28.3375, 1.5) -> (-28.3375, 3)
  line L15 (-28.337, 1.5) -> (-6.3413, 1.5)
  line L16 (230.642, -112.3) -> (230.642, -113.3)
  line L17 (230.642, -113.3) -> (222.602, -113.3)
  line L18 (-36.12, -117.7958) -> (-31.338, -117.8)
  line L19 (222.602, -113.3) -> (222.602, -112.3)
  line L20 (-28.337, -113.3) -> (-28.337, -112.3)
  line L21 (-29.3375, -113.3) -> (-29.338, -113.3)
  arc A2 (-38.6178, -115.2937) -> (-36.12, -117.7958) centre (-36.1178, -115.2958) ccw
  line L22 (57.336, -112.3) -> (-20.297, -112.3)
  line L23 (8.02, 1) -> (8.02, 0)
  line L24 (-29.3375, -112.3) -> (-29.3375, -113.3)
  line L25 (-33.0995, -112.3) -> (-33.0995, 1.5)
  line L26 (-29.338, -112.3) -> (-33.0995, -112.3)
  line L27 (57.336, -113.3) -> (57.336, -112.3)
  line L28 (-20.297, -113.3) -> (-28.337, -113.3)
  line L29 (-29.338, -113.3) -> (-29.338, -112.3)
  line L30 (-20.297, -112.3) -> (-20.297, -113.3)
  line L31 (301.275, 5.5) -> (-36.0995, 5.5)
  line L32 (-38.5995, -94.25) -> (-38.6178, -115.2937)
  line L33 (298.2751, -76.2) -> (298.2751, -93.25)
  line L34 (298.275, -95.25) -> (298.275, -95.25)
  line L35 (298.275, -76.2) -> (298.275, -76.2)
  line L36 (-6.3413, 1.5) -> (-6.3413, 0)
  line L37 (-38.5995, 3) -> (-38.5995, -94.25)
  arc A3 (303.775, 3) -> (301.275, 5.5) centre (301.275, 3) ccw
  line L38 (298.2751, -74.2) -> (298.275, -74.2)
  line L39 (-28.337, 3) -> (-28.337, 1.5)
  line L40 (-33.0995, 1.5) -> (-28.3375, 1.5)
  line L41 (-0.02, 0) -> (-0.02, 1)
  arc A4 (-36.0995, 5.5) -> (-38.5995, 3) centre (-36.0995, 3) ccw
  line L42 (-31.338, -117.8) -> (302.0217, -117.8)
  line L43 (-6.3413, 0) -> (-0.02, 0)
  line L44 (298.275, -57.15) -> (298.275, -57.15)
  line L45 (-0.02, 1) -> (8.02, 1)
  line L46 (8.02, 0) -> (171.43, 0)
  line L47 (-28.3375, 3) -> (-28.337, 3)
  line L48 (290.235, 0) -> (290.235, 1)
  line L49 (290.235, 1) -> (298.275, 1)
  line L50 (298.2751, -57.15) -> (298.2751, -74.2)
  line L51 (298.275, 1) -> (298.275, -57.15)
  line L52 (222.602, -112.3) -> (65.376, -112.3)
  line L53 (-33.0995, -112.3) -> (-33.0995, 1.5)
  line L54 (301.275, 5.5) -> (-36.0995, 5.5)
  line L55 (-31.338, -117.8) -> (302.0217, -117.8)
  line L56 (57.336, -112.3) -> (-20.297, -112.3)
  line L57 (8.02, 0) -> (171.43, 0)
  line L58 (290.2351, -112.3) -> (230.642, -112.3)
  line L59 (298.2751, -95.25) -> (298.2751, -113.3)
  line L60 (298.275, -76.2) -> (298.275, -76.2)
  line L61 (298.275, -74.2) -> (298.275, -76.2)
  line L62 (298.2751, -76.2) -> (298.2751, -93.25)
  line L63 (298.2751, -93.25) -> (298.275, -93.25)
  line L64 (298.275, -93.25) -> (298.275, -95.25)
  line L65 (290.2351, -113.3) -> (290.2351, -112.3)
  arc A5 (302.0217, -117.8) -> (304.5217, -115.3) centre (302.0374, -115.3157) ccw
  line L66 (179.47, 0) -> (290.235, 0)
  line L67 (298.2751, -113.3) -> (290.2351, -113.3)
  line L68 (304.5217, -115.3) -> (303.775, 3)
  line L69 (298.275, -95.25) -> (298.275, -95.25)
  line L70 (57.336, -113.3) -> (57.336, -112.3)
  line L71 (65.376, -113.3) -> (57.336, -113.3)
  line L72 (-29.338, -113.3) -> (-29.338, -112.3)
  line L73 (-6.3413, 1.5) -> (-6.3413, 0)
  line L74 (-29.3375, -113.3) -> (-29.338, -113.3)
  line L75 (-29.3375, -112.3) -> (-29.3375, -113.3)
  line L76 (-28.3375, 1.5) -> (-28.3375, 3)
  line L77 (-28.337, 1.5) -> (-6.3413, 1.5)
  line L78 (-28.337, -112.3) -> (-29.3375, -112.3)
  line L79 (-28.337, -113.3) -> (-28.337, -112.3)
  line L80 (-28.3375, 3) -> (-28.337, 3)
  line L81 (-20.297, -113.3) -> (-28.337, -113.3)
  line L82 (65.376, -112.3) -> (65.376, -113.3)
  line L83 (-20.297, -112.3) -> (-20.297, -113.3)
  line L84 (-29.338, -112.3) -> (-33.0995, -112.3)
  line L85 (8.02, 1) -> (8.02, 0)
  line L86 (-28.337, 3) -> (-28.337, 1.5)
  arc A6 (-38.6178, -115.2937) -> (-36.12, -117.7958) centre (-36.1178, -115.2958) ccw
  line L87 (-38.5995, -94.25) -> (-38.6178, -115.2937)
  line L88 (-38.5995, 3) -> (-38.5995, -94.25)
  line L89 (-0.02, 0) -> (-0.02, 1)
  line L90 (-33.0995, 1.5) -> (-28.3375, 1.5)
  line L91 (-6.3413, 0) -> (-0.02, 0)
  arc A7 (-36.0995, 5.5) -> (-38.5995, 3) centre (-36.0995, 3) ccw
  line L92 (-0.02, 1) -> (8.02, 1)
  line L93 (-36.12, -117.7958) -> (-31.338, -117.8)
  line L94 (298.275, -93.25) -> (298.275, -95.25)
  line L95 (298.2751, -113.3) -> (290.2351, -113.3)
  line L96 (290.2351, -113.3) -> (290.2351, -112.3)
  line L97 (298.2751, -93.25) -> (298.275, -93.25)
  line L98 (298.275, -74.2) -> (298.275, -76.2)
  line L99 (298.2751, -74.2) -> (298.275, -74.2)
  line L100 (290.235, 0) -> (290.235, 1)
  line L101 (179.47, 1) -> (179.47, 0)
  line L102 (230.642, -113.3) -> (222.602, -113.3)
  line L103 (179.47, 1) -> (179.47, 0)
  line L104 (171.43, 1) -> (179.47, 1)
  line L105 (222.602, -112.3) -> (65.376, -112.3)
  line L106 (65.376, -112.3) -> (65.376, -113.3)
  line L107 (65.376, -113.3) -> (57.336, -113.3)
  line L108 (171.43, 0) -> (171.43, 1)
  line L109 (171.43, 1) -> (179.47, 1)
  line L110 (125.838, -2.5) -> (125.838, -0.5)
  line L111 (125.838, -0.5) -> (-32.5995, -0.5)
  line L112 (-32.5995, -0.5) -> (-32.5995, -111.8)
  line L113 (-32.5995, -111.8) -> (297.7751, -111.8)
  line L114 (297.775, -111.8) -> (297.7751, -0.5)
  line L115 (297.7751, -0.5) -> (139.338, -0.5)
  line L116 (139.338, -0.5) -> (139.338, -2.5)
  line L117 (139.338, -2.5) -> (295.7751, -2.5)
  line L118 (295.7751, -2.5) -> (295.7751, -109.8)
  line L119 (295.7751, -109.8) -> (-30.5995, -109.8)
  line L120 (-30.5995, -109.8) -> (-30.5995, -2.5)
  line L121 (-30.5995, -2.5) -> (125.838, -2.5)
  line L122 (-27.837, -112.3) -> (-27.837, -112.8)
  line L123 (-27.837, -112.8) -> (-20.797, -112.8)
  line L124 (-20.797, -112.3) -> (-20.797, -112.8)
  line L125 (-20.797, -112.3) -> (-20.797, -111.8)
  line L126 (-27.837, -112.3) -> (-27.837, -111.8)
  dimension "d61" = 5.5
  dimension "d62" = 5.5
  dimension "d63" = 6.2339
  dimension "d64" = 5.5125
  dimension "d65" = 5.5
  dimension "d66" = 6.2276
  dimension "d67" = 5.5188
  dimension "d89" = 0.5
  dimension "d90" = 0.5
  constraint coincident L5.start L8.start
  constraint perpendicular L0 L8
  constraint coincident L8.end L59
  constraint coincident L4.end L7.start
  constraint perpendicular L7 L48
  constraint coincident L7.end L51
  constraint perpendicular L28 L122
  constraint perpendicular L83 L123
  constraint perpendicular L123 L124
  constraint coincident L113 L125.end
  constraint perpendicular L113 L125
  constraint coincident L113 L126.end
  constraint perpendicular L113 L126
  measures "d61" distance of L42 L58
  measures "d62" distance of L4 L31
  measures "d63" distance of L0.end L3
  measures "d64" distance of L1.start L3
  measures "d65" distance of L25 L37
  measures "d66" distance of L8.end L3
  measures "d67" distance of L7.end L68
  measures "d89" distance of L13.start L122.start
  measures "d90" distance of L22.end L124.start
equation "d84 = ( 330.375 / 2 ) * 1 mm"
equation "d85 = ( 13.5 / 2 ) * 1 mm"
